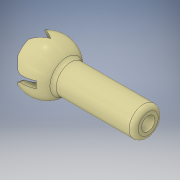
# Autodesk Inventor part: Castor
Saved by Autodesk Inventor 2016 (Build 200138000, 138)
## iProperties
Created: 2016-10-13
Part Number: Castor
Material: Generic
Document SubType Name: Modeling
Designer: desirw
Density: 1 g/cm^3
Appearance: Default
Author: desirw
Autodesk Inventor part; units mm, degrees
ref_plane "Work Plane1" through (8.7249, 0, 0) normal (1, 0, 0) x (0, 1, 0)
sketch "Sketch2" plane through (8.7249, 0, 0) normal (1, 0, 0) x (0, 1, 0)
  circle A0 centre (0, 0) radius 6.477
  dimension "d21" = 12.954
  constraints: 1 centre point, 1 coincident
  measures "d21" diameter of A0
extrude "OUter Shell" add sketch "Sketch2" along normal blind 44.6278
sketch "Sketch3" plane through (8.7249, 0, 0) normal (-1, 0, 0) x (0, 0, 1)
  arc A0 (11.176, 0) -> (-11.176, 0) centre (0, 0) ccw
  line L0 (-11.176, 0) -> (11.176, 0)
  dimension "d57" = 22.352
  constraints: 2 end point, 2 point on circle, 1 centre point, 1 coincident, 1 horizontal
  measures "d57" distance of L0.start L0.end
revolve "Revolution2" add sketch "Sketch3" angle 360 about axis through (8.7249, 0, -11.176) along (0, 0, 1)
ref_plane "Work Plane8" through (5.5499, 0, 0) normal (1, 0, 0) x (0, 1, 0)
sketch "Sketch5" plane through (5.5499, 0, 0) normal (1, 0, 0) x (0, 1, 0)
  arc A0 (0, 9.5352) -> (0, -9.5352) centre (0, 0) ccw
  line L0 (0, 9.5352) -> (0, -9.5352)
  dimension "d12" = 19.0703
  constraints: 2 end point, 2 point on circle, 1 centre point, 1 coincident, 1 vertical
  measures "d12" diameter of A0
revolve "Inner Shell" cut sketch "Sketch5" angle 360 about axis through (5.5499, 0, 9.5352) along (0, 0, -1)
ref_plane "Work Plane9" through (0, 0, 11.1125) normal (0, 0, 1) x (1, 0, 0)
sketch "Sketch7" plane through (0, 0, 11.1125) normal (0, 0, 1) x (1, 0, 0)
  ellipse E0 centre (3.175, 0) end of major axis (3.175, 5.4125) minor radius 3.3411
  point P0 (0, 0)
  constraints: 2 other
extrude "Oval Expansion" cut sketch "Sketch7" against normal blind 25.4
sketch "Sketch8" plane through (53.3527, 0, 0) normal (1, 0, 0) x (0, 0, -1)
  circle A0 centre (0, 0) radius 2.9972
  dimension "d20" = 5.9944
  constraints: 1 centre point, 1 coincident
  measures "d20" diameter of A0
ref_plane "Work Plane15" through (39.3954, 0, 0) normal (1, 0, 0) x (0, 1, 0)
sketch "Sketch10" plane through (39.3954, 0, 0) normal (1, 0, 0) x (0, 1, 0)
  circle A0 centre (0, 0) radius 2.8702
  dimension "d29" = 5.7404
  constraints: 1 centre point, 1 coincident
  measures "d29" diameter of A0
extrude "Extrusion4" cut sketch "Sketch10" against normal blind 3.81
sketch "Sketch12" plane through (0, 0, 0) normal (0, 0, 1) x (1, 0, 0)
  line L0 (6.096, 1.524) -> (13.716, 1.524)
  line L1 (13.716, 1.524) -> (13.716, -1.524)
  line L2 (13.716, -1.524) -> (6.096, -1.524)
  line L3 (6.096, -1.524) -> (6.096, 1.524)
  point P0 (0, 0)
  dimension "d39" = 7.62
  constraints: 8 end point, 2 parallel, 1 horizontal, 1 perpendicular
  measures "d39" distance of L1.end L2.end
extrude "Extrusion6" cut sketch "Sketch12" along normal through all both and the other way through all
ref_plane "Work Plane12" through (37.0332, 0, 0) normal (1, 0, 0) x (0, 1, 0)
sketch "Sketch13" plane through (37.0332, 0, 0) normal (1, 0, 0) x (0, 1, 0)
  circle A0 centre (0, 0) radius 2.8702
  dimension "d41" = 5.7404
  constraints: 1 centre point, 1 coincident
  measures "d41" diameter of A0
loft "Loft2" cut profiles "Sketch8" section 2 edges at (35.5854, -2.8702, 0)
sketch "Sketch14" plane through (37.0332, 0, 0) normal (1, 0, 0) x (0, 1, 0)
  circle A0 centre (0, 0) radius 2.54
  dimension "d46" = 5.08
  constraints: 1 centre point, 1 coincident
  measures "d46" diameter of A0
extrude "Extrusion7" add sketch "Sketch13" against normal blind 12.7
extrude "Extrusion8" cut sketch "Sketch14" against normal blind 12.7
sketch "Sketch17" plane through (0, 0, 11.1125) normal (0, 0, 1) x (1, 0, 0)
  line L0 (1.7856, 4.9223) -> (1.7856, 8.7607) projected
  line L1 (17.8327, -6.477) -> (17.8327, 6.477) projected
  line L2 (1.7856, 14.6236) -> (17.761, 14.6236)
  line L3 (9.7733, 14.6236) -> (9.7733, -12.9972)
  line L4 (1.7856, -8.7607) -> (1.7856, -4.9223) projected
  line L5 (1.7856, 8.7607) -> (9.7733, 0.1249)
  line L6 (9.7733, 0.1249) -> (1.7856, -8.7607)
  point P0 (0, 0)
  dimension "d60" = 16.047
  constraints: 8 end point, 1 coincident, 1 horizontal, 1 midpoint, 1 point on line, 1 vertical
  measures "d60" distance between parallel lines of L0 L1
sketch "Sketch18" plane through (0, 0, 0) normal (0, 0, 1) x (1, 0, 0)
  line L0 (1.7856, 4.9223) -> (1.7856, 8.7607) projected
  line L1 (5.4659, 0.0659) -> (1.7856, 8.7607)
  line L2 (1.7856, 8.7607) -> (1.7856, -8.7607)
  arc A0 (1.7856, -8.7607) -> (1.7856, 8.7607) centre (5.5499, 0) ccw projected
  line L3 (1.7856, -8.7607) -> (1.7856, -4.9223) projected
  line L4 (5.4659, 0.0659) -> (1.7856, -8.7607)
  point P0 (0, 0)
  constraints: 6 end point, 1 collinear, 1 point on circle
sketch "Sketch19" plane through (0, 0, 0) normal (0, 1, 0) x (-1, 0, 0)
  line L0 (-10.1859, 0) -> (-2.5311, 0) construction
  line L1 (-10.1859, 0) -> (-3.9661, 0) construction
  line L2 (-10.1859, 0) -> (-3.0039, 0) construction
  line L3 (-10.1859, 0) -> (-0.3588, 5.6737)
  line L4 (-10.1859, 0) -> (1.1615, 0) construction
  line L5 (-0.3588, 5.6737) -> (-0.3588, -5.6737)
  line L6 (-10.1859, 0) -> (-0.3588, -5.6737)
  line L7 (-10.1859, 0) -> (0.1303, 0) construction
  point P0 (0, 0)
  dimension "d65" = 30
  dimension "d66" = 30
  constraints: 16 end point, 5 horizontal, 1 equal length, 1 vertical
  measures "d65" angle of L4 L3
  measures "d66" angle of L6 L7
extrude "Extrusion10" cut sketch "Sketch19" along normal mid plane 25.4
pattern_circular "Circular Pattern1" count 4 over 360 about axis through (8.7249, 0, 0) along (1, 0, 0) of "Extrusion10"
fillet "Fillet1" radius 2.54 1 edges at (17.8327, -6.477, 0)
fillet "Fillet2" radius 2.032 1 edges at (53.3527, -6.477, 0)
chamfer "Chamfer1" distance 1.27 angle 45 8 edges at (3.9893, -5.2493, -7.8057) (3.9893, -5.2493, 7.8057) (5.1126, 4.4094, 8.443) (2.4579, 5.2864, 7.3084) (2.4579, 5.2864, -7.3084) (5.1126, 4.4094, -8.443) (5.918, -3.0903, -9.013) (5.918, -3.0903, 9.013)
chamfer "Chamfer2" distance 2.54 angle 45 4 edges at (1.7856, 6.6891, 5.6574) (1.7856, -6.6891, 5.6574) (1.7856, -6.6891, -5.6574) (1.7856, 6.6891, -5.6574)
body "Solid1"
